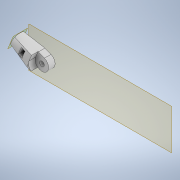
# Autodesk Inventor part: Hangar
Saved by Autodesk Inventor 2021 (Build 250183000, 183)
## iProperties
Created: 2020-10-20
Part Number: Hangar
Material: Generic
Document SubType Name: Modeling
Designer: VM
Density: 1 g/cm^3
Appearance: Default
Author: VM
Autodesk Inventor part; units mm, degrees
note: some values were not read from the file. Chosen so that the rebuilt part matches the saved one: direction of "Hole1".
ref_plane "YZ Plane" through (0, 0, 0) normal (1, 0, 0) x (0, 1, 0)
ref_plane "XZ Plane" through (0, 0, 0) normal (0, 1, 0) x (-1, 0, 0)
ref_plane "XY Plane" through (0, 0, 0) normal (0, 0, 1) x (1, 0, 0)
ref_plane "Work Plane1" through (0, 0, 0) normal (0, 0, 1) x (1, 0, 0)
sketch "Sketch1" plane through (0, 0, 0) normal (0, 0, 1) x (1, 0, 0)
  circle A0 centre (-15, -15) radius 1.2
  circle A1 centre (-89, -15) radius 1.2
  circle A2 centre (-89, -15) radius 1.75
  line L0 (-89, -15) -> (-112.137643, -5.443064) construction
  line L1 (-87.137402, -10.359731) -> (-91.777544, -8.497184)
  line L2 (-95.50274, -17.777722) -> (-90.862598, -19.640269)
  arc A3 (-90.862598, -19.640269) -> (-87.137402, -10.359731) centre (-89, -15) ccw
  line L3 (-95.50274, -17.777722) -> (-91.777544, -8.497184)
  point P0 (-100.568822, -10.221532)
  dimension "d1" = 3.5
  dimension "d10" = 5
  constraints: 10 end point, 2 centre point, 2 parallel, 2 point on circle, 2 tangent, 1 coincident, 1 midpoint
  measures "d1" diameter of A2
  measures "d10" distance of L2.start L2.end
extrude "Extrusion1" add sketch "Sketch1" along normal blind 10 contours A3 L2 L3 L1
ref_plane "Work Plane2" through (-109.423166, -12.19008, 0) normal (-0.9280284, 0.3725094, 0) x (0, 0, 1)
sketch "Sketch3" plane through (-109.423166, -12.19008, 0) normal (-0.9280284, 0.3725094, 0) x (0, 0, 1)
  line L0 (0, 10.000274) -> (0, 0)
  line L1 (0, 0) -> (10, 0)
  line L2 (10, 10.000274) -> (10, 0)
  line L3 (0, 10.000274) -> (10, 10.000274)
  circle A0 centre (4.999863, 5.000137) radius 5.000137
  point P0 (0, 52.073903)
  constraints: 3 tangent, 1 centre point
sketch "Sketch3 outline for Loft1" plane through (-109.423166, -12.19008, 0) normal (-0.9280284, 0.3725094, 0) x (0, 0, 1)
  circle A0 centre (4.999863, 5.000137) radius 5.000137
loft "Loft1" add profiles "Sketch3 outline for Loft1" section 2 edges at (-93.640142, -13.137453, 0) (-95.50274, -17.777722, 5) (-93.640142, -13.137453, 10) (-91.777544, -8.497184, 5)
sketch "Sketch5" plane through (0, 0, 10) normal (0, 0, 1) x (1, 0, 0)
  circle A0 centre (-89, -15) radius 5.25
  arc A1 (-90.862598, -19.640269) -> (-87.137402, -10.359731) centre (-89, -15) ccw
  point P0 (0, 0)
  dimension "d18" = 10.5
  constraints: 1 centre point, 1 concentric
  measures "d18" diameter of A0
extrude "Extrusion3" cut sketch "Sketch5" against normal blind 5
sketch "Sketch6" plane through (0, 0, 10) normal (0, 0, 1) x (1, 0, 0)
  line L0 (-99.397863, -14.059118) -> (-102.181949, -12.94159)
  line L1 (-102.181949, -12.94159) -> (-99.946892, -7.373419)
  line L2 (-99.946892, -7.373419) -> (-97.162807, -8.490948)
  line L3 (-97.162807, -8.490948) -> (-99.397863, -14.059118)
  line L4 (-116.544319, -29.930925) -> (-85.605283, 47.147132)
  line L5 (-95.50274, -17.777722) -> (-92.347771, -19.044123)
  point P0 (0, 0)
  dimension "d21" = 7
  dimension "d22" = 3
  dimension "d23" = 6
  dimension "d24" = 2
  constraints: 8 end point, 3 perpendicular, 1 parallel
  measures "d21" distance between parallel lines of L4 L1
  measures "d22" distance of L0.start L0.end
  measures "d23" distance of L2.end L0.start
  measures "d24" distance between parallel lines of L5 L0
extrude "Extrusion4" cut sketch "Sketch6" against normal blind 9
sketch "Sketch7" plane through (-107.560568, -7.549811, 4.999863) normal (-0.9280284, 0.3725094, 0) x (0, 0, 1)
  arc A0 (-3.535582, -3.535679) -> (3.535582, -3.535679) centre (0, 0) ccw
  point P0 (-4.999863, 47.073766)
  constraints: 1 coincident
hole "Hole1" at (-107.560568, -7.549811, 4.999863) direction (0.9280284, -0.3725094, 0) diameter 3.5 depth 7
sketch "Sketch8" plane through (0, 0, 10) normal (0, 0, 1) x (1, 0, 0)
  line L0 (-88.622575, -9.763584) -> (-91.777544, -8.497184)
  arc A0 (-88.622575, -9.763584) -> (-93.043836, -11.651883) centre (-89, -15) ccw
  spline S0 degree 2 poles (-93.872149, -13.044325) (-93.566724, -12.283424) (-93.043836, -11.651883) knots 0 0 0 1 1 1 weights 1 0.98802352 1
  line L1 (-93.872149, -13.044325) -> (-92.009551, -8.404056)
  arc A1 (-88.622575, -9.763584) -> (-92.347771, -19.044123) centre (-89, -15) ccw
  line L2 (-92.009551, -8.404056) -> (-88.622575, -9.763584)
  point P0 (0, 0)
  constraints: 4 end point, 1 collinear, 1 perpendicular, 1 other
extrude "Extrusion5" cut sketch "Sketch8" against normal blind 5
body "Solid1"
